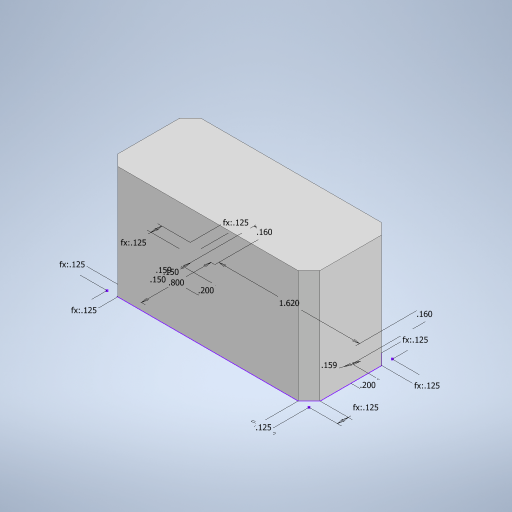
# Autodesk Inventor part: Servo Mount and Screw Hole Test
Saved by Autodesk Inventor 2023 (Build 270158000, 158)
## iProperties
Created: 2023-03-13
Part Number: Servo Mount and Screw Hole Test
Material: Generic
Document SubType Name: Modeling
Designer: tommy
Density: 1 g/cm^3
Appearance: Default
Author: tommy
Autodesk Inventor part; units mm, degrees
ref_plane "YZ Plane" through (0, 0, 0) normal (1, 0, 0) x (0, 1, 0)
ref_plane "XZ Plane" through (0, 0, 0) normal (0, 1, 0) x (-1, 0, 0)
ref_plane "XY Plane" through (0, 0, 0) normal (0, 0, 1) x (1, 0, 0)
sketch "Sketch1" plane through (0, 0, 0) normal (0, 1, 0) x (-1, 0, 0)
  line L0 (0, 0) -> (41.148, 0)
  line L1 (41.148, 0) -> (41.148, -20.32)
  line L2 (41.148, -20.32) -> (0, -20.32)
  line L3 (0, -20.32) -> (0, 0)
  line L4 (47.498, 2.0259) -> (-5.588, 2.0259)
  line L5 (-5.588, -22.3459) -> (47.1979, -22.3459)
  circle A0 centre (45.212, -15.24) radius 2.0193
  circle A1 centre (-4.064, -15.24) radius 2.0193
  line L6 (41.148, -10.16) -> (50.3729, -10.16)
  line L7 (41.148, -13.97) -> (50.3729, -13.97)
  line L8 (41.148, -6.35) -> (50.3729, -6.35)
  line L9 (0, -10.16) -> (-8.7354, -10.16)
  line L10 (-5.588, 2.0259) -> (-5.5604, 2.0259)
  line L11 (-8.7354, -1.1491) -> (-8.7354, -19.1709)
  line L12 (-5.5604, -22.3459) -> (-5.588, -22.3459)
  line L13 (47.498, -22.3459) -> (47.1979, -22.3459)
  line L14 (50.3729, -19.1709) -> (50.3729, -1.1491)
  line L15 (47.1979, 2.0259) -> (47.498, 2.0259)
  circle A2 centre (45.212, -5.08) radius 2.0193
  circle A3 centre (-4.064, -5.08) radius 2.0193
  line L16 (-5.5604, 2.0259) -> (-8.7354, -1.1491)
  line L17 (-8.7354, -19.1709) -> (-5.5604, -22.3459)
  line L18 (47.1979, -22.3459) -> (50.3729, -19.1709)
  line L19 (50.3729, -1.1491) -> (47.1979, 2.0259)
  point P0 (41.148, -6.35)
  point P1 (41.148, -13.97)
  point P2 (-8.7354, 2.0259)
  point P3 (-8.7354, -22.3459)
  point P4 (50.3729, -22.3459)
  point P5 (50.3729, 2.0259)
  point P6 (46.7819, -6.35)
  point P7 (43.6421, -6.35)
  point P8 (43.6421, -13.97)
  point P9 (46.7819, -13.97)
  dimension "d0" = 41.148
  dimension "d1" = 20.32
  dimension "d4" = 4.0386
  dimension "d5" = 4.0386
  dimension "d6" = 3.81
  dimension "d7" = 3.81
  dimension "d16" = 5.08
  dimension "d17" = 5.08
  dimension "d18" = 4.064
  dimension "d19" = 4.064
  dimension "d20" = 3.175
  dimension "d21" = 3.175
  dimension "d22" = 3.175
  dimension "d23" = 3.175
  dimension "d24" = 3.175
  dimension "d25" = 3.175
  dimension "d26" = 3.175
  dimension "d27" = 3.175
  constraints: 40 end point, 12 point on line, 5 parallel, 5 perpendicular, 4 centre point, 4 midpoint, 2 horizontal, 2 symmetric about line, 2 other
  measures "d0" distance of L1.end L2.end
  measures "d1" distance of L0.end L1.end
  measures "d4" diameter of A0
  measures "d5" diameter of A1
  measures "d6" distance between parallel lines of L6 L7
  measures "d7" distance between parallel lines of L6 L8
  measures "d16" distance from line of L6 A0.centre
  measures "d17" distance from line of L9 A1.centre
  measures "d18" distance from line of L1 A0.centre
  measures "d19" distance from line of L3 A1.centre
  measures "d20" distance of L10.end point (-8.735, 2.026)
  measures "d21" distance of L11.start point (-8.735, 2.026)
  measures "d22" distance of L11.end point (-8.735, -22.346)
  measures "d23" distance of L12.start point (-8.735, -22.346)
  measures "d24" distance of L5.end point (50.373, -22.346)
  measures "d25" distance of L14.start point (50.373, -22.346)
  measures "d26" distance of L14.end point (50.373, 2.026)
  measures "d27" distance of L15.start point (50.373, 2.026)
extrude "Extrusion1" add sketch "Sketch1" along normal blind 33.02 contours L3 L9 L11 L16 L4 L19 L14 L8 A2 L1 L0 | L0 L1 L2 L3 | L3 L2 L1 L7 A0 L14 L18 L5 L17 L11 L9 | L8 A2 L14 L6 L1 | L6 L14 L7 A0 L1 | A2 L8 | L8 A2 | L7 A0 | A0 L7 | A1 | A3
extrude "Extrusion2" cut sketch "Sketch1" along normal blind 24.638 contours L7 A0 | A0 L7 | A1
extrude "Extrusion3" cut sketch "Sketch1" along normal blind 29.845 contours L0 L1 L2 L3
extrude "Extrusion4" cut sketch "Sketch1" along normal up to surface (24.638 mm away) contours L8 A2 L14 L6 L1 | L6 L14 L7 A0 L1 | A2 L8 | L8 A2 | A3
equation "\"d21\" = d20"
equation "\"d22\" = d20"
equation "\"d23\" = d22"
equation "\"d24\" = d20"
equation "\"d25\" = d24"
equation "\"d26\" = d20"
equation "\"d27\" = d26"
body "Solid1"
